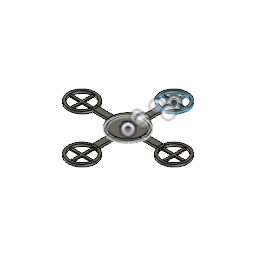
drone (Autodesk Fusion 360 design; units mm, degrees)
part number: 2026-03-05-10-47-19-794
Autodesk Fusion 360 part; units mm, degrees
sketch "Sketch1" plane through (0, 0, 0) normal (0, 0, 1) x (1, 0, 0)
  circle A0 centre (0, 200) radius 50
  circle A1 centre (0, 200) radius 60
  circle A2 centre (0, 0) radius 75
  circle A3 centre (0, 0) radius 75
  circle A4 centre (0, 0) radius 65
  line L0 (-25, 65) -> (0, 65)
  line L1 (-25, 150) -> (25, 150)
  line L2 (5, 255.05) -> (-5, 255.05)
  line L3 (-5, 255.05) -> (-5, 144.95)
  line L4 (-5, 144.95) -> (5, 144.95)
  line L5 (5, 144.95) -> (5, 255.05)
  line L6 (5, 255.05) -> (-5, 144.95) construction
  line L7 (-5, 255.05) -> (5, 144.95) construction
  line L8 (55.05, 195) -> (-55.05, 195)
  line L9 (-55.05, 195) -> (-55.05, 205)
  line L10 (-55.05, 205) -> (55.05, 205)
  line L11 (55.05, 205) -> (55.05, 195)
  line L12 (55.05, 195) -> (-55.05, 205) construction
  line L13 (-55.05, 195) -> (55.05, 205) construction
  point P0 (0, 200)
  point P1 (0, 200)
  dimension "d2" = 100
  dimension "d3" = 10
  dimension "d6" = 150
  dimension "d7" = 0
  dimension "d11" = 25
  dimension "d12" = 200
  dimension "d15" = 85
  dimension "d16" = 10
  dimension "d17" = 110.1
  dimension "d18" = 110.1
  dimension "d19" = 10
  constraint coincident A2.centre A3.centre
  constraint horizontal L0
  constraint tangent A4 L0
  constraint horizontal L2
  constraint perpendicular L2 L3
  constraint parallel L2 L4
  constraint parallel L3 L5
  constraint coincident L6 P1
  constraint coincident L7 P1
  constraint coincident P0 A0.centre
  constraint horizontal L8
  constraint perpendicular L8 L9
  constraint parallel L8 L10
  constraint parallel L9 L11
  constraint coincident L12 P1
  constraint coincident L13 P1
  constraint coincident P1 P0
  measures "d2" diameter of A0
  measures "d6" diameter of A2
  measures "d11" distance of L0.start L0.end
  measures "d12" distance of P0 A2.centre
  measures "d15" distance of L0.start L1.start
  measures "d16" distance of L3.end L4.end
  measures "d17" distance of L2.end L3.end
  measures "d18" distance of L9.end L10.end
  measures "d19" distance of L8.end L9.end
extrude "Extrude1" add sketch "Sketch1" along normal blind 5 contours A0 L5 L8 L10 | A0 L3 L5 L10 | L3 L5 L8 L10 | A0 L3 L5 L8 | A0 L3 L8 L10 makes body 1
sketch "Sketch2" plane through (0, 0, 0) normal (0, 0, 1) x (1, 0, 0)
  line L0 (0, 150) -> (0, 65)
  line L1 (0, 65) -> (0, 107.5)
  line L2 (0, 150) -> (12.5, 150)
  line L3 (12.5, 150) -> (12.5, 65)
  line L4 (12.5, 65) -> (0, 65)
  line L5 (0, 65) -> (0, 150)
  line L6 (0, 150) -> (-12.5, 150)
  line L7 (-12.5, 150) -> (-12.5, 65)
  line L8 (-12.5, 65) -> (0, 65)
  line L9 (0, 65) -> (0, 150)
  dimension "d23" = 85
  dimension "d24" = 42.5
  dimension "d25" = 12.5
  dimension "d26" = 85
  dimension "d27" = 85
  dimension "d28" = 12.5
  constraint vertical L0
  constraint parallel L0 L1
  constraint horizontal L2
  constraint vertical L3
  constraint horizontal L4
  constraint vertical L5
  constraint horizontal L6
  constraint vertical L7
  constraint horizontal L8
  constraint vertical L9
  measures "d23" distance of L0.start L0.end
  measures "d24" distance of L0.end L1.end
  measures "d25" distance of L0.start L2.end
  measures "d26" distance of L0.start L0.end
  measures "d27" distance of L0.start L0.end
  measures "d28" distance of L0.start L6.end
extrude "Extrude2" add sketch "Sketch1" along normal blind 10 separate body contours A0 L8 L10 L11 | A0 L2 L3 L5 | L1 L3 L4 L5 | A0 L8 L9 L10 | A1 makes body 2
extrude "Extrude3" add sketch "Sketch2" along normal blind 10 separate body makes body 3
extrude "Extrude4" add sketch "Sketch1" along normal blind 5 separate body contours A4 makes body 4
extrude "Extrude5" add sketch "Sketch1" along normal blind 10 separate body contours A2 A3 makes body 5
sketch "Sketch3" plane through (0, 0, 0) normal (0, 0, 1) x (1, 0, 0)
pattern_circular "C-Pattern1" count 4 over 360 about axis through (0, 0, 1.75) along (0, 0, 1) of bodies 2 1 3 makes body 6 at (-180, 0, 0) makes body 7 at (0, -180, 0) makes body 8 at (180, 0, 0) makes body 9 at (-197.0092, 59.9254, 6.6667) makes body 10 at (-59.9254, -197.0092, 6.6667) makes body 11 at (197.0092, -59.9254, 6.6667) makes body 12 at (-121.6667, -8.3333, 0) makes body 13 at (8.3333, -121.6667, 0) makes body 14 at (121.6667, 8.3333, 0)
other "Base Mesh Feature1"
other "Scale1"
sketch "Sketch4" plane through (0, 0, 5) normal (0, 0, 1) x (-1, 0, 0)
  line L0 (-5, -205) -> (-5, -249.7494)
  arc A0 (-5, -249.7494) -> (5, -249.7494) centre (0, -200) ccw
  line L1 (5, -249.7494) -> (5, -205)
  line L2 (5, -205) -> (49.7494, -205)
  arc A1 (49.7494, -205) -> (49.7494, -195) centre (0, -200) ccw
  line L3 (49.7494, -195) -> (5, -195)
  line L4 (5, -195) -> (5, -150.2506)
  arc A2 (5, -150.2506) -> (-5, -150.2506) centre (0, -200) ccw
  line L5 (-5, -150.2506) -> (-5, -195)
  line L6 (-5, -195) -> (-49.7494, -195)
  arc A3 (-49.7494, -195) -> (-49.7494, -205) centre (0, -200) ccw
  line L7 (-49.7494, -205) -> (-5, -205)
  point P0 (0, -200)
  constraint coincident P0 A0.centre
other "Scale2"
other "Modify1"
other "Modify2"
sketch "Sketch5" plane through (0, 0, 0) normal (0, 1, 0) x (1, 0, 0)
equation "outer_rotor_diameter = 100 mm"
equation "d2 = outer_rotor_diameter"
equation "d3 = outer_ring_thickness"
equation "outer_ring_thickness = 10 mm"
equation "center_platform_diameter = 150 mm"
equation "d6 = center_platform_diameter"
equation "center_platform_border_thickness = 10 mm"
equation "d9 = -center_platform_border_thickness"
equation "arm_width = 25 mm"
equation "d11 = arm_width"
equation "d12 = center_to_center"
equation "center_to_center = 200 mm"
equation "arm_length = center_to_center - 0.5 * outer_rotor_diameter - 0.5 * center_platform_diameter + outer_ring_thickness"
equation "d15 = arm_length"
equation "d16 = outer_rotor_diameter * 0.1"
equation "d17 = outer_rotor_diameter + outer_ring_thickness + 0.1 mm"
equation "d18 = outer_ring_thickness + 0.1 mm + outer_rotor_diameter"
equation "d19 = outer_rotor_diameter * 0.1"
equation "rotor_cross_height = 5 mm"
equation "d21 = rotor_cross_height"
equation "d24 = arm_length / 2"
equation "d25 = arm_width / 2"
equation "d26 = arm_length"
equation "d27 = arm_length"
equation "d28 = arm_width / 2"
equation "platform_inner_thickess = 5 mm"
equation "platform_border_thickness = 10 mm"
equation "rotor_border_thickness = 10 mm"
equation "d32 = rotor_border_thickness"
equation "arm_thickness = 10 mm"
equation "d35 = arm_thickness"
equation "d37 = platform_inner_thickess"
equation "d39 = center_platform_border_thickness"
